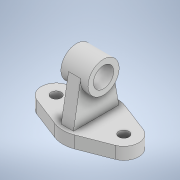
# Autodesk Inventor part: ShaftSupport
Saved by Autodesk Inventor 2022.2 (Build 262287030, 287C)
## iProperties
Created: 2023-04-14
Part Number: ShaftSupport
Material: Generic
Document SubType Name: Modeling
Designer: jak27277
Mass: 222.533 g
Surface Area: 395.769 cm^2
Volume: 222.533 cm^3
Density: 1 g/cm^3
Appearance: Default
Author: jak27277
Autodesk Inventor part; units mm, degrees
ref_plane "YZ Plane" through (0, 0, 0) normal (1, 0, 0) x (0, 1, 0)
ref_plane "XZ Plane" through (0, 0, 0) normal (0, 1, 0) x (-1, 0, 0)
ref_plane "XY Plane" through (0, 0, 0) normal (0, 0, 1) x (1, 0, 0)
sketch "Sketch1" plane through (0, 0, 0) normal (0, 1, 0) x (-1, 0, 0)
  line L0 (50, 0) -> (-50, 0) construction
  line L1 (50, 22) -> (-50, 22)
  line L2 (-50, -22) -> (50, -22)
  arc A0 (50, -22) -> (50, 22) centre (50, 0) ccw
  arc A1 (-50, 22) -> (-50, -22) centre (-50, 0) ccw
  circle A2 centre (50, 0) radius 7.5
  circle A3 centre (-50, 0) radius 7.5
  line L3 (57.92, 20.525) -> (14.4, 37.3181)
  line L4 (-14.4, 37.3181) -> (-57.92, 20.525)
  line L5 (0, 0) -> (0, 42.8746) construction
  arc A4 (14.4, 37.3181) -> (-14.4, 37.3181) centre (0, 0) ccw
  line L6 (57.92, -20.525) -> (14.4, -37.3181)
  line L7 (-14.4, -37.3181) -> (-57.92, -20.525)
  line L8 (0, 0) -> (0, -42.8746) construction
  arc A5 (-14.4, -37.3181) -> (14.4, -37.3181) centre (0, 0) ccw
  point P0 (-57.92, -20.525)
  dimension "d0" = 100
  dimension "d1" = 40
  dimension "d2" = 15
  dimension "d3" = 22
  constraints: 20 end point, 10 point on circle, 8 tangent, 6 centre point, 5 symmetric about line, 4 coincident, 4 point on line, 1 equal radius, 1 horizontal, 1 midpoint, 1 parallel, 1 vertical, 1 other
  measures "d0" distance of L0.start L0.end
  measures "d1" radius of A4
  measures "d2" diameter of A2
  measures "d3" radius of A0
extrude "Extrusion1" add sketch "Sketch1" along normal blind 18
sketch "Sketch2" plane through (0, 0, 0) normal (1, 0, 0) x (0, 1, 0)
  line L0 (0, 0) -> (76, 0) construction
  circle A0 centre (76, 0) radius 23
  circle A1 centre (76, 0) radius 15
  line L1 (18, -20.525) -> (18, -37.3181) construction
  line L2 (18, -37.3181) -> (18, -37.3181) construction
  line L3 (18, -37.3181) -> (18, -20.525) construction
  line L4 (18, -20.525) -> (18, 20.525) construction
  line L5 (18, 20.525) -> (18, 37.3181) construction
  line L6 (18, 37.3181) -> (18, 37.3181) construction
  line L7 (18, 37.3181) -> (18, 20.525) construction
  line L8 (18, 20.525) -> (18, -20.525) construction
  line L9 (18, 7.5) -> (18, -7.5) construction
  line L10 (18, 7.5) -> (18, -7.5) construction
  line L11 (79.9649, -22.6557) -> (18, -33.5)
  line L12 (79.9649, 22.6557) -> (18, 33.5)
  line L13 (18, -33.5) -> (18, 33.5)
  point P0 (79.9649, 22.6557)
  point P1 (18, 0)
  dimension "d8" = 46
  dimension "d7" = 67
  dimension "d9" = 30
  dimension "d14" = 116
  constraints: 8 end point, 2 symmetric about line, 1 centre point, 1 coincident, 1 collinear, 1 horizontal, 1 midpoint, 1 point on line, 4 other
  measures "d7" distance of L12.end L11.end
  measures "d9" diameter of A1
  measures "d14" diameter of L0.end point (18, 0)
extrude "Extrusion2" add sketch "Sketch2" along normal mid plane 18
extrude "Extrusion3" add sketch "Sketch2" along normal mid plane 40 contours A0
body "Solid1"
